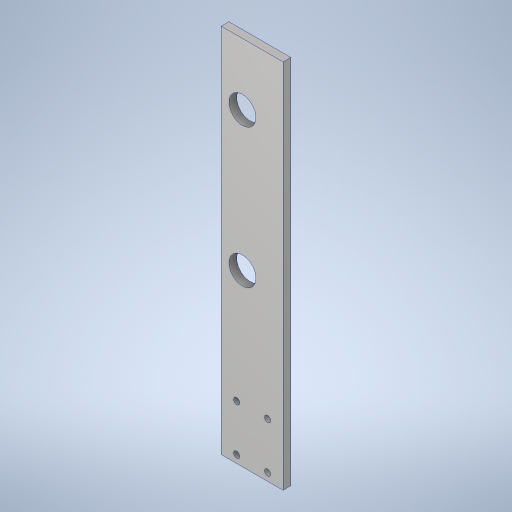
# Autodesk Inventor part: GP1-002
Saved by Autodesk Inventor 2023.4 (Build 274418000, 418)
## iProperties
Created: 2025-01-05
Part Number: GP1-002
Material: Aluminum 6061
Document SubType Name: Modeling
Designer: mavericks
Density: 2.7 g/cm^3
Appearance: Aluminum - Flat
Author: mavericks
Autodesk Inventor part; units mm, degrees
ref_plane "YZ Plane" through (0, 0, 0) normal (1, 0, 0) x (0, 1, 0)
ref_plane "XZ Plane" through (0, 0, 0) normal (0, 1, 0) x (-1, 0, 0)
ref_plane "XY Plane" through (0, 0, 0) normal (0, 0, 1) x (1, 0, 0)
sketch "Sketch1" plane through (0, 0, 0) normal (0, 0, 1) x (1, 0, 0)
  line L0 (-25.4, 152.4) -> (25.4, 152.4)
  line L1 (25.4, 152.4) -> (25.4, -152.4)
  line L2 (25.4, -152.4) -> (-25.4, -152.4)
  line L3 (-25.4, -152.4) -> (-25.4, 152.4)
  line L4 (-25.4, 152.4) -> (25.4, -152.4) construction
  line L5 (25.4, 152.4) -> (-25.4, -152.4) construction
  circle A0 centre (-7.9375, -12.7) radius 25.4 construction
  circle A1 centre (-7.9375, -12.7) radius 11.1125
  circle A2 centre (-7.9375, -12.7) radius 38.1 construction
  circle A3 centre (-7.9375, -12.7) radius 50.8 construction
  circle A4 centre (-7.9375, 101.6) radius 25.4 construction
  circle A5 centre (-7.9375, 101.6) radius 11.1125
  circle A6 centre (-7.9375, 101.6) radius 38.1 construction
  circle A7 centre (-7.9375, 101.6) radius 50.8 construction
  point P0 (0, 0)
  dimension "d0" = 50.8
  dimension "d1" = 304.8
  dimension "d3" = 50.8
  dimension "d4" = 22.225
  dimension "d7" = 17.4625
  dimension "d8" = 76.2
  dimension "d9" = 101.6
  dimension "d10" = 50.8
  dimension "d11" = 22.225
  dimension "d12" = 76.2
  dimension "d13" = 101.6
  dimension "d14" = 114.3
  dimension "d15" = 139.7
  constraints: 12 end point, 8 centre point, 6 coincident, 2 midpoint, 2 parallel, 1 horizontal, 1 perpendicular, 1 vertical alignment
  measures "d0" distance of L1.end L2.end
  measures "d1" distance of L0.end L1.end
  measures "d3" diameter of A0
  measures "d4" diameter of A1
  measures "d7" distance from line of L3 A1.centre
  measures "d8" diameter of A2
  measures "d9" diameter of A3
  measures "d10" diameter of A4
  measures "d11" diameter of A5
  measures "d12" diameter of A6
  measures "d13" diameter of A7
  measures "d14" distance of A0.centre A4.centre
  measures "d15" distance from line of L2 A0.centre
extrude "Extrusion1" add sketch "Sketch1" along normal blind 6.35
sketch "Sketch2" plane through (0, 0, 6.35) normal (0, 0, 1) x (1, 0, 0)
  line L0 (-25.4, 152.4) -> (-25.4, -152.4) construction
  line L1 (-12.7, -107.95) -> (12.7, -107.95) construction
  line L2 (-25.4, -152.4) -> (25.4, -152.4) construction
  point P0 (0, 0)
  point P1 (-12.7, -146.05)
  point P2 (12.7, -146.05)
  point P3 (0, -107.95)
  dimension "d19" = 25.4
  dimension "d21" = 38.1
  dimension "d22" = 6.35
  constraints: 3 vertical alignment, 2 end point, 2 horizontal alignment, 1 horizontal, 1 midpoint
  measures "d19" distance of L1.end L1.start
  measures "d21" distance of point (-12.7, -146.05) L1.start
  measures "d22" distance from line of L2 point (-12.7, -146.05)
hole "Hole1" at (-12.7, -107.95, 6.35) at (12.7, -107.95, 6.35) at (-12.7, -146.05, 6.35) at (12.7, -146.05, 6.35) direction (0, 0, -1) diameter 5.1054 end through all clearance for "Flat Head Machine Screw (82)" size "#10" standard "Ansi Unified Screw Threads"
body "Solid1"
